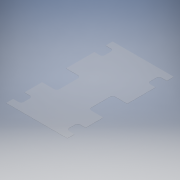
# Autodesk Inventor part: Belly Pan
Saved by Autodesk Inventor 2019.4 (Build 234330000, 330)
## iProperties
Created: 2019-12-14
Part Number: Belly Pan
Material: Polycarbonate, Clear
Document SubType Name: Modeling
Designer: Mark
Density: 1.2 g/cm^3
Appearance: Polycarbonate - Clear
Mass: 1324.8 g
Surface Area: 7435.6 cm^2
Volume: 1104 cm^3
Author: Mark
Autodesk Inventor part; units mm, degrees
ref_plane "YZ Plane" through (0, 0, 0) normal (1, 0, 0) x (0, 1, 0)
ref_plane "XZ Plane" through (0, 0, 0) normal (0, 1, 0) x (-1, 0, 0)
ref_plane "XY Plane" through (0, 0, 0) normal (0, 0, 1) x (1, 0, 0)
sketch "Sketch1" plane through (0, 0, 0) normal (0, 1, 0) x (-1, 0, 0)
  line L0 (-230, 400) -> (230, 400)
  line L1 (230, 400) -> (230, -400)
  line L2 (230, -400) -> (-230, -400)
  line L3 (-230, -400) -> (-230, 400)
  line L4 (-230, 400) -> (230, -400) construction
  line L5 (230, 400) -> (-230, -400) construction
  point P0 (0, 0)
  dimension "d0" = 460
  dimension "d1" = 800
  constraints: 12 end point, 2 midpoint, 2 parallel, 1 horizontal, 1 perpendicular
  measures "d0" distance of L1.end L2.end
  measures "d1" distance of L0.end L1.end
extrude "Extrusion1" add sketch "Sketch1" along normal blind 2
sketch "Sketch2" plane through (0, 2, 0) normal (0, 1, 0) x (1, 0, 0)
  line L0 (-230, 400) -> (-230, -400) projected
  line L1 (-230, -130) -> (-120, -130)
  line L2 (-120, -130) -> (-120, 50)
  line L3 (-120, 50) -> (-230, 50)
  line L4 (-230, 50) -> (-230, -130)
  line L5 (230, 400) -> (-230, 400) projected
  line L6 (230, -130) -> (120, -130)
  line L7 (120, -130) -> (120, 50)
  line L8 (120, 50) -> (230, 50)
  line L9 (230, 50) -> (230, -130)
  line L10 (230, -400) -> (230, 400) projected
  line L11 (-230, -40) -> (230, -40) construction
  line L12 (-230, -40) -> (230, -40) construction
  line L13 (-230, -347.5) -> (-170, -347.5)
  line L14 (-170, -347.5) -> (-170, -262.5)
  line L15 (-170, -262.5) -> (-230, -262.5)
  line L16 (-230, -262.5) -> (-230, -347.5)
  line L17 (-230, -400) -> (230, -400) projected
  line L18 (0, -400) -> (0, -300) construction
  line L19 (0, -400) -> (100, -400) construction
  line L20 (230, -347.5) -> (170, -347.5)
  line L21 (170, -347.5) -> (170, -262.5)
  line L22 (170, -262.5) -> (230, -262.5)
  line L23 (230, -262.5) -> (230, -347.5)
  line L24 (-230, 182.5) -> (-230, 267.5)
  line L25 (-230, 347.5) -> (-170, 347.5)
  line L26 (-170, 347.5) -> (-170, 262.5)
  line L27 (-170, 262.5) -> (-230, 262.5)
  line L28 (-230, 262.5) -> (-230, 347.5)
  line L29 (230, 347.5) -> (170, 347.5)
  line L30 (170, 347.5) -> (170, 262.5)
  line L31 (170, 262.5) -> (230, 262.5)
  line L32 (230, 262.5) -> (230, 347.5)
  point P0 (0, 0)
  dimension "d4" = 110
  dimension "d5" = 180
  dimension "d6" = 350
  dimension "d7" = 110
  dimension "d8" = 180
  dimension "d9" = 350
  dimension "d12" = 460
  dimension "d13" = 0
  dimension "d14" = 60
  dimension "d15" = 85
  dimension "d16" = 222.5
  dimension "d17" = 100
  dimension "d18" = 90
  dimension "d19" = 60
  dimension "d20" = 85
  dimension "d21" = 52.5
  dimension "d22" = 60
  dimension "d23" = 85
  dimension "d24" = 52.5
  constraints: 58 end point, 10 parallel, 7 horizontal, 6 perpendicular, 6 symmetric about line, 4 point on line, 2 equal length, 2 midpoint, 1 collinear, 1 vertical
  measures "d4" distance of L3.end L2.end
  measures "d5" distance of L2.end L1.end
  measures "d6" distance between parallel lines of L5 L3
  measures "d7" distance of L7.end L8.end
  measures "d8" distance of L6.end L7.end
  measures "d9" distance between parallel lines of L5 L8
  measures "d12" distance of L11.start L11.end
  measures "d13" distance between parallel lines of L12 L11
  measures "d14" distance of L15.end L14.end
  measures "d15" distance of L14.end L13.end
  measures "d16" distance between parallel lines of L11 L15
  measures "d17" distance of L18.start L18.end
  measures "d18" angle of L19 L18
  measures "d19" distance of L26.end L27.end
  measures "d20" distance of L25.end L26.end
  measures "d21" distance between parallel lines of L5 L25
  measures "d22" distance of L31.end L30.end
  measures "d23" distance of L30.end L29.end
  measures "d24" distance between parallel lines of L5 L29
extrude "Extrusion2" cut sketch "Sketch2" against normal blind 3 contours L25 L26 L27 L0 | L10 L31 L30 L29 | L9 L6 L7 L8 | L3 L2 L1 L0 | L10 L20 L21 L22 | L15 L14 L13 L0
fillet "Fillet1" radius 20 12 edges at (120, 1, 130) (120, 1, -50) (170, 1, 262.5) (170, 1, 347.5) (170, 1, -262.5) (170, 1, -347.5) (-170, 1, 347.5) (-170, 1, 262.5) (-120, 1, 130) (-120, 1, -50) (-170, 1, -262.5) (-170, 1, -347.5)
body "Solid1"
